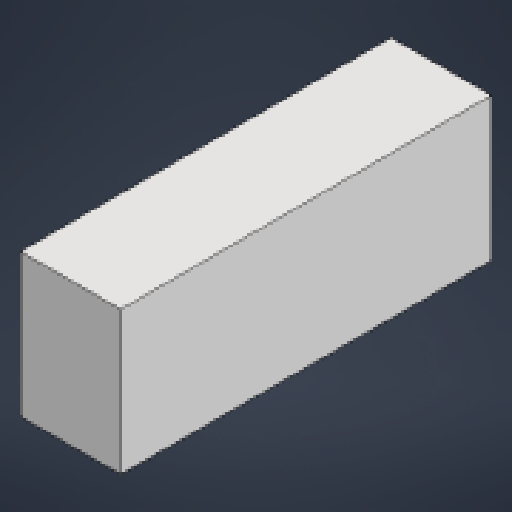
# Autodesk Inventor part: 3DPRINT,LIMIT_SWITCH,SPACER,RIGHT
Saved by Autodesk Inventor 2026.1 (Build 301233020, 233B)
## iProperties
Created: 2026-02-01
Part Number: 3DPRINT,LIMIT_SWITCH,SPACER,RIGHT
Material: ABS Plastic
Document SubType Name: Modeling
Designer: Owen L
Mass: 3.84326 g
Surface Area: 21.9106 cm^2
Volume: 3.62572 cm^3
Density: 1.06 g/cm^3
Appearance: Smooth - Black
Author: Owen L
Autodesk Inventor part; units mm, degrees
ref_plane "YZ Plane" through (0, 0, 0) normal (1, 0, 0) x (0, 1, 0)
ref_plane "XZ Plane" through (0, 0, 0) normal (0, 1, 0) x (-1, 0, 0)
ref_plane "XY Plane" through (0, 0, 0) normal (0, 0, 1) x (1, 0, 0)
sketch "Sketch1" plane through (0, 0, 0) normal (1, 0, 0) x (0, 1, 0)
  line L0 (6.1, 15.8) -> (-6.1, 15.8)
  line L1 (-6.1, 15.8) -> (-6.1, -15.8)
  line L2 (-6.1, -15.8) -> (6.1, -15.8)
  line L3 (6.1, -15.8) -> (6.1, 15.8)
  line L4 (6.1, 15.8) -> (-6.1, -15.8) construction
  line L5 (-6.1, 15.8) -> (6.1, -15.8) construction
  line L6 (1.0374, 8.001) -> (1.0374, -8.001) construction
  line L7 (3.1837, 8.001) -> (3.1837, -8.001)
  line L8 (-1.1089, -8.001) -> (-1.1089, 8.001)
  arc A0 (3.1837, 8.001) -> (-1.1089, 8.001) centre (1.0374, 8.001) ccw
  arc A1 (-1.1089, -8.001) -> (3.1837, -8.001) centre (1.0374, -8.001) ccw
  point P0 (0, 0)
  point P1 (1.0374, 0)
  dimension "d0" = 12.2
  dimension "d1" = 31.6
  dimension "d4" = 7.1374
  dimension "d5" = 16.002
  dimension "d6" = 4.2926
  constraints: 20 end point, 4 point on circle, 4 tangent, 3 midpoint, 3 parallel, 2 centre point, 1 horizontal, 1 horizontal alignment, 1 perpendicular, 1 vertical
  measures "d0" distance of L2.end L1.end
  measures "d1" distance of L1.end L0.end
  measures "d4" distance between parallel lines of L1 L6
  measures "d5" distance of L6.start L6.end
  measures "d6" distance between parallel lines of L7 L8
extrude "Extrusion1" add sketch "Sketch1" along normal blind 12
fillet "Fillet1" radius 0.5 4 edges at (6, -6.1, 15.8) (6, 6.1, 15.8) (6, 6.1, -15.8) (6, -6.1, -15.8)
body "Solid1"
